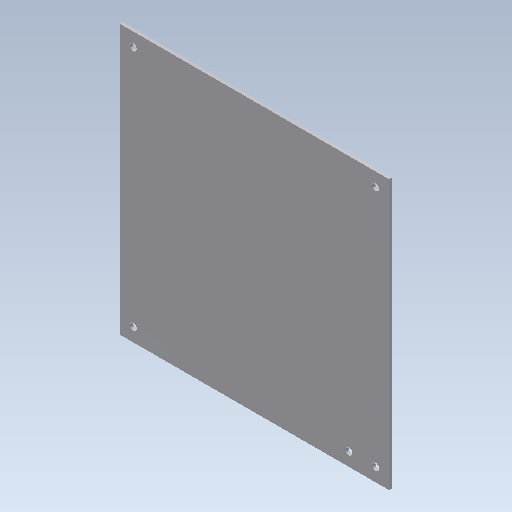
# Autodesk Inventor part: 5-HOLE DIFFUSOR_INSIDE FLY BUBBLE
Saved by Autodesk Inventor 2020.3 (Build 243373000, 373)
## iProperties
RuleStatus: InUse
AfterDocSave0: file://Part Number Cleaner
Created: 2014-06-24
Material: Generic
Vendor: HHMI: JFRC - ID&F
Document SubType Name: Modeling
Designer: NEGRASHOVI
Density: 1 g/cm^3
Appearance: Snow
DESIGN DEPARTMENT: HHMI: JFRC - ID&F
ALTERED ITEM PART NUMBER: 2447
ALTERED ITEM VENDOR: OPTIX
ALTERED ITEM DESCRIPTION: N/A
Author: NEGRASHOVI
Revision Number: 0
Autodesk Inventor part; units mm, degrees
ref_plane "YZ Plane" through (0, 0, 0) normal (1, 0, 0) x (0, 1, 0)
ref_plane "XZ Plane" through (0, 0, 0) normal (0, 1, 0) x (-1, 0, 0)
ref_plane "XY Plane" through (0, 0, 0) normal (0, 0, 1) x (1, 0, 0)
sketch "Sketch1" plane through (0, 0, 0) normal (0, 0, 1) x (1, 0, 0)
  line L0 (-127, -127) -> (127, -127)
  line L1 (127, -127) -> (127, 127)
  line L2 (127, 127) -> (-127, 127)
  line L3 (-127, 127) -> (-127, -127)
  line L4 (-127, -127) -> (127, 127) construction
  point P0 (0, 0)
  point P1 (0, 0)
  dimension "d0" = 254
  dimension "d1" = 254
  constraints: 10 end point, 2 parallel, 1 coincident, 1 horizontal, 1 midpoint, 1 perpendicular
  measures "d0" distance of L1.end L2.end
  measures "d1" distance of L2.end L0.start
extrude "Extrusion1" add sketch "Sketch1" along normal blind 3
sketch "Sketch2" plane through (0, 0, 3) normal (0, 0, 1) x (1, 0, 0)
  line L0 (-114.3, -114.3) -> (114.3, -114.3) construction
  line L1 (114.3, -114.3) -> (114.3, 114.3) construction
  line L2 (114.3, 114.3) -> (-114.3, 114.3) construction
  line L3 (-114.3, 114.3) -> (-114.3, -114.3) construction
  line L4 (-114.3, -114.3) -> (114.3, 114.3) construction
  point P0 (0, 0)
  point P1 (0, 0)
  point P2 (88.9, -114.3)
  dimension "d4" = 228.6
  dimension "d5" = 228.6
  constraints: 10 end point, 5 coincident, 2 parallel, 1 horizontal, 1 midpoint, 1 perpendicular, 1 point on line
  measures "d4" distance of L2.end L0.start
  measures "d5" distance of L1.end L2.end
hole "Hole1" at (-114.3, 114.3, 3) at (114.3, 114.3, 3) at (114.3, -114.3, 3) at (-114.3, -114.3, 3) direction (0, 0, -1) diameter 6.7564 end through all
sketch "Sketch3" plane through (0, 0, 3) normal (0, 0, 1) x (1, 0, 0)
  point P0 (0, 0)
  point P1 (88.9, -114.3)
hole "Hole2" at (88.9, -114.3, 3) direction (0, 0, -1) diameter 6.7564 depth 25.4 tip angle 118
body "Solid1"
